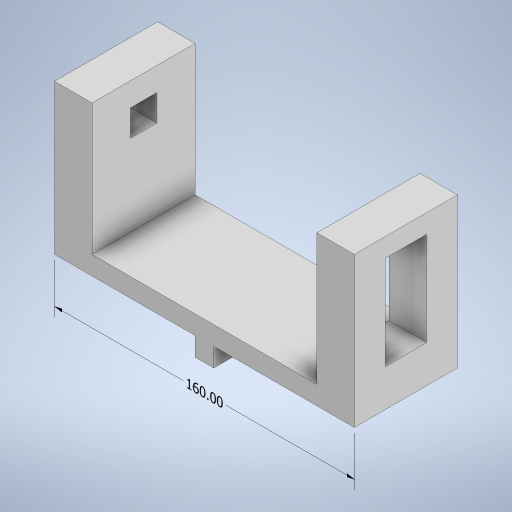
# Autodesk Inventor part: camera_support
Saved by Autodesk Inventor 2023 (Build 270158000, 158)
## iProperties
Created: 2022-07-03
Part Number: camera_support
Material: Genérico
Document SubType Name: Modeling
Designer: inigo
Density: 1 g/cm^3
Appearance: Valor por defecto
Author: inigo
Autodesk Inventor part; units mm, degrees
ref_plane "YZ Plane" through (0, 0, 0) normal (1, 0, 0) x (0, 1, 0)
ref_plane "XZ Plane" through (0, 0, 0) normal (0, 1, 0) x (-1, 0, 0)
ref_plane "XY Plane" through (0, 0, 0) normal (0, 0, 1) x (1, 0, 0)
sketch "Boceto1" plane through (0, 0, 0) normal (0, 0, 1) x (1, 0, 0)
  line L0 (-80, 5) -> (80, 5)
  line L1 (80, 5) -> (80, -5)
  line L2 (80, -5) -> (-80, -5)
  line L3 (-80, -5) -> (-80, 5)
  line L4 (-80, 5) -> (80, -5) construction
  line L5 (80, 5) -> (-80, -5) construction
  point P0 (0, 0)
  dimension "d0" = 160
  dimension "d1" = 10
  constraints: 12 end point, 2 midpoint, 2 parallel, 1 horizontal, 1 perpendicular
  measures "d0" distance of L1.end L2.end
  measures "d1" distance of L0.end L1.end
extrude "Extrusión1" add sketch "Boceto1" along normal blind 55
sketch "Boceto2" plane through (-80, 5, 0) normal (0, 1, 0) x (1, 0, 0)
  line L0 (0, 0) -> (0, -55) projected
  line L1 (0, -55) -> (160, -55) projected
  line L2 (0, 0) -> (20, 0)
  line L3 (20, 0) -> (20, -55)
  line L4 (20, -55) -> (0, -55)
  line L5 (0, -55) -> (0, 0)
  line L6 (160, 0) -> (160, -55) projected
  line L7 (160, 0) -> (140, 0)
  line L8 (140, 0) -> (140, -55)
  line L9 (140, -55) -> (160, -55)
  line L10 (160, -55) -> (160, 0)
  point P0 (80, 0)
  dimension "d4" = 20
  dimension "d5" = 20
  constraints: 16 end point, 4 parallel, 2 horizontal, 2 perpendicular, 2 point on line
  measures "d4" distance of L3.end L4.end
  measures "d5" distance of L9.end L8.end
extrude "Extrusión2" add sketch "Boceto2" along normal blind 70
sketch "Boceto3" plane through (-80, -5, 0) normal (-1, 0, 0) x (0, 0, 1)
  line L0 (0, 80) -> (55, 80) projected
  line L1 (20.5, 67.5) -> (34.5, 67.5)
  line L2 (34.5, 67.5) -> (34.5, 53.5)
  line L3 (34.5, 53.5) -> (20.5, 53.5)
  line L4 (20.5, 53.5) -> (20.5, 67.5)
  line L5 (20.5, 67.5) -> (34.5, 53.5) construction
  line L6 (34.5, 67.5) -> (20.5, 53.5) construction
  line L7 (0, 0) -> (0, 80) projected
  point P0 (0, 5)
  point P1 (27.5, 60.5)
  dimension "d10" = 14
  dimension "d11" = 14
  dimension "d12" = 20.5
  dimension "d13" = 12.5
  constraints: 12 end point, 2 midpoint, 2 parallel, 1 horizontal, 1 perpendicular
  measures "d10" distance of L2.end L3.end
  measures "d11" distance of L1.end L2.end
  measures "d12" distance between parallel lines of L7 L4
  measures "d13" distance between parallel lines of L0 L1
extrude "Extrusión3" cut sketch "Boceto3" against normal blind 70
sketch "Boceto4" plane through (-80, -5, 0) normal (0, -1, 0) x (1, 0, 0)
  line L0 (140, 55) -> (20, 55) projected
  line L1 (75, 25) -> (85, 25)
  line L2 (85, 25) -> (85, 55)
  line L3 (85, 55) -> (75, 55)
  line L4 (75, 55) -> (75, 25)
  line L5 (75, 25) -> (85, 55) construction
  line L6 (85, 25) -> (75, 55) construction
  point P0 (80, 0)
  dimension "d17" = 10
  dimension "d30" = 30
  constraints: 12 end point, 2 parallel, 1 horizontal, 1 perpendicular, 1 point on line
  measures "d17" distance of L3.end L2.end
  measures "d30" distance between parallel lines of L1 L0
extrude "Extrusión4" add sketch "Boceto4" along normal blind 10
sketch "Boceto5" plane through (80, -5, 55) normal (1, 0, 0) x (0, 0, -1)
  line L0 (0, 80) -> (55, 80) projected
  line L1 (55, 0) -> (55, 80) projected
  line L2 (16.5, 20) -> (16.5, 70)
  line L3 (16.5, 70) -> (38.5, 70)
  line L4 (38.5, 70) -> (38.5, 20)
  line L5 (38.5, 20) -> (16.5, 20)
  line L6 (16.5, 20) -> (38.5, 70) construction
  line L7 (16.5, 70) -> (38.5, 20) construction
  line L8 (0, 0) -> (0, 80) projected
  point P0 (55, 5)
  point P1 (27.5, 45)
  point P2 (16.5, 45)
  dimension "d26" = 50
  dimension "d27" = 22
  dimension "d28" = 16.5
  dimension "d29" = 10
  constraints: 12 end point, 3 midpoint, 2 parallel, 1 perpendicular
  measures "d26" distance of L3.end L4.end
  measures "d27" distance of L2.end L3.end
  measures "d28" distance from line of L8 point (16.5, 45)
  measures "d29" distance between parallel lines of L3 L0
extrude "Extrusión5" cut sketch "Boceto5" against normal blind 30
